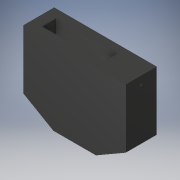
# Autodesk Inventor part: HA01
Saved by Autodesk Inventor 2017 (Build 210142000, 142)
## iProperties
Created: 2018-10-18
Part Number: HA01
Material: ABS Plastic
Document SubType Name: Modeling
Designer: Dell
Density: 1.06 g/cm^3
Appearance: Smooth - Black
Author: Dell
Autodesk Inventor part; units mm, degrees
ref_plane "YZ Plane" through (0, 0, 0) normal (1, 0, 0) x (0, 1, 0)
ref_plane "XZ Plane" through (0, 0, 0) normal (0, 1, 0) x (-1, 0, 0)
ref_plane "XY Plane" through (0, 0, 0) normal (0, 0, 1) x (1, 0, 0)
sketch "Sketch1" plane through (0, 0, 0) normal (0, 0, 1) x (1, 0, 0)
  line L0 (0, -144.3376) -> (-125, -72.1688)
  line L1 (-125, -72.1688) -> (-125, 72.1688)
  line L2 (-125, 72.1688) -> (0, 144.3376) construction
  line L3 (0, 144.3376) -> (125, 72.1688) construction
  line L4 (125, 72.1688) -> (125, -72.1688)
  line L5 (125, -72.1688) -> (0, -144.3376)
  line L6 (125, 72.1688) -> (-125, 72.1688)
  line L7 (125, 72.1688) -> (-125, 72.1688)
  line L8 (-125, 72.1688) -> (-125, 144.3376)
  line L9 (-125, 144.3376) -> (125, 144.3376)
  line L10 (125, 144.3376) -> (125, 72.1688)
  point P0 (0, 0)
  point P1 (0, 0)
  dimension "d0" = 250
  constraints: 22 end point, 2 horizontal, 2 parallel, 2 vertical alignment, 1 coincident, 1 midpoint, 1 perpendicular, 13 other
  measures "d0" distance between parallel lines of L4 L1
extrude "Extrusion1" add sketch "Sketch1" along normal blind 75 contours L0 L1 L6 L4 L5
sketch "Sketch2" plane through (-125, 72.1688, 0) normal (0, 1, 0) x (1, 0, 0)
  line L0 (175, -55) -> (25, -55)
  line L1 (25, -55) -> (25, -20)
  line L2 (25, -20) -> (175, -20)
  line L3 (175, -20) -> (175, -55)
  line L4 (200, 0) -> (0, 0)
  line L5 (0, 0) -> (0, -75)
  point P0 (100, 0)
  point P1 (100, -20)
  point P2 (100, 0)
  point P3 (25, -37.5)
  point P4 (0, -37.5)
  dimension "d3" = 150
  dimension "d4" = 35
  constraints: 12 end point, 4 midpoint, 2 parallel, 1 horizontal, 1 horizontal alignment, 1 perpendicular, 1 vertical alignment
  measures "d3" distance of L0.start L0.end
  measures "d4" distance of L0.end L1.end
extrude "Extrusion2" cut sketch "Sketch2" against normal through all
sketch "Sketch3" plane through (0, 0, 75) normal (0, 0, 1) x (1, 0, 0)
  line L0 (125, -114.3376) -> (-125, -114.3376)
  line L1 (-125, -114.3376) -> (-125, -144.3376)
  line L2 (-125, -144.3376) -> (125, -144.3376)
  line L3 (125, -144.3376) -> (125, -114.3376)
  point P0 (0, 0)
  point P1 (0, -144.3376)
  point P2 (0, -114.3376)
  point P3 (125, -72.1688)
  dimension "d7" = 30
  constraints: 8 end point, 2 parallel, 2 vertical alignment, 1 horizontal, 1 horizontal alignment, 1 midpoint, 1 perpendicular
  measures "d7" distance of L2.end L0.start
extrude "Extrusion3" cut sketch "Sketch3" against normal through all
sketch "Sketch4" plane through (125, -72.1688, 0) normal (1, 0, 0) x (0, 0, -1)
  circle A0 centre (-37.5, 124.3376) radius 3
  line L0 (0, 144.3376) -> (-75, 144.3376) projected
  point P0 (-37.5, 144.3376)
  dimension "d14" = 6
  dimension "d15" = 20
  constraints: 1 centre point, 1 midpoint, 1 vertical alignment
  measures "d14" diameter of A0
  measures "d15" distance from line of L0 A0.centre
extrude "Extrusion4" cut sketch "Sketch4" against normal through all
body "Solid1"
